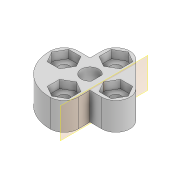
# Autodesk Inventor part: sonic hub 1_4 D 3mm
Saved by Autodesk Inventor 2020 (Build 240168000, 168)
## iProperties
Created: 2019-12-14
Part Number: sonic hub 1_4 D 3mm
Material: Generic
Document SubType Name: Modeling
Designer: ball
Density: 1 g/cm^3
Appearance: Default
Author: ball
Autodesk Inventor part; units mm, degrees
ref_plane "YZ Plane" through (0, 0, 0) normal (1, 0, 0) x (0, 1, 0)
ref_plane "XZ Plane" through (0, 0, 0) normal (0, 1, 0) x (-1, 0, 0)
ref_plane "XY Plane" through (0, 0, 0) normal (0, 0, 1) x (1, 0, 0)
sketch "Sketch1" plane through (0, 0, 0) normal (0, 1, 0) x (-1, 0, 0)
  circle A0 centre (9.779, 0) radius 1.9304
  line L0 (0, 9.779) -> (0, 0) construction
  line L1 (9.779, 0) -> (0, 0) construction
  arc A1 (-2.5908, -2.0472) -> (-2.5908, 2.0472) centre (0, 0) ccw
  line L2 (-2.5908, 2.0472) -> (-2.5908, -2.0472)
  circle A2 centre (0, 9.779) radius 1.9304
  circle A3 centre (-9.779, 0) radius 1.9304
  circle A4 centre (0, -9.779) radius 1.9304
  line L3 (4.7625, 7.21) -> (-2.8575, 7.21) construction
  line L4 (-2.8575, 7.21) -> (-2.8575, 3.81) construction
  line L5 (-2.8575, 3.81) -> (4.7625, 3.81) construction
  line L6 (4.7625, 3.81) -> (4.7625, 7.21) construction
  line L7 (4.7625, 8.2835) -> (7.5625, 8.2835) construction
  line L8 (7.5625, 8.2835) -> (7.5625, 2.3835) construction
  line L9 (7.5625, 2.3835) -> (4.7625, 2.3835) construction
  line L10 (4.7625, 2.3835) -> (4.7625, 8.2835) construction
  circle A5 centre (0, -9.779) radius 5.2959 construction
  circle A6 centre (0, 9.779) radius 5.2959 construction
  circle A7 centre (9.779, 0) radius 5.2959 construction
  circle A8 centre (-9.779, 0) radius 5.2959 construction
  line L11 (-5.2959, 9.779) -> (-5.2959, -11.9726) construction
  line L12 (-9.779, 5.2959) -> (-5.2959, 5.2959)
  line L13 (-13.5238, -3.7448) -> (-3.7448, -13.5238)
  line L14 (5.2959, -9.779) -> (5.2959, 9.779) construction
  line L15 (9.779, -5.2959) -> (5.2959, -5.2959)
  line L16 (5.2959, -9.779) -> (5.2959, -5.2959)
  arc A9 (-9.779, 5.2959) -> (-13.5238, -3.7448) centre (-9.779, 0) ccw
  arc A10 (-3.7448, -13.5238) -> (5.2959, -9.779) centre (0, -9.779) ccw
  line L17 (-5.2959, 9.779) -> (-5.2959, 5.2959)
  arc A11 (15.0749, 0) -> (0, 15.0749) centre (0, 0) ccw
  arc A12 (0, 15.0749) -> (-5.2959, 9.779) centre (0, 9.779) ccw
  arc A13 (9.779, -5.2959) -> (15.0749, 0) centre (9.779, 0) ccw
  dimension "d0" = 3.8608
  dimension "d2" = 0
  dimension "d3" = 9.779
  dimension "d12" = 6.604
  dimension "d13" = 2.5908
  dimension "d16" = 360
  dimension "d18" = 7.62
  dimension "d19" = 3.4
  dimension "d20" = 3.81
  dimension "d21" = 2.8
  dimension "d22" = 5.9
  dimension "d23" = 10.5918
  dimension "d24" = 10.5918
  dimension "d25" = 10.5918
  dimension "d26" = 10.5918
  constraints: 36 end point, 22 point on circle, 14 centre point, 10 coincident, 8 tangent, 4 parallel, 4 perpendicular, 3 point on line, 3 vertical, 2 collinear, 2 concentric, 2 horizontal, 9 other
  measures "d0" diameter of A0
  measures "d2" vertical distance of L0.end A0.centre
  measures "d3" distance of L0.end A0.centre
  measures "d12" diameter of A1
  measures "d13" distance from line of L2 L0.end
  measures "d18" distance of L5.end L4.end
  measures "d19" distance of L4.end L3.end
  measures "d20" distance from line of L0.end L5
  measures "d21" distance of L8.end L9.end
  measures "d22" distance of L7.end L8.end
  measures "d23" diameter of A5
  measures "d24" diameter of A6
  measures "d25" diameter of A7
  measures "d26" diameter of A8
extrude "Extrusion1" add sketch "Sketch1" along normal mid plane 10.4
sketch "Sketch2" plane through (0, 5.2, 0) normal (0, 1, 0) x (1, 0, 0)
  circle A0 centre (-9.779, 0) radius 1.9304 construction
  circle A1 centre (-9.779, 0) radius 4.6609 construction
  line L0 (-14.4399, 0) -> (-12.1095, 4.0365)
  line L1 (-12.1095, 4.0365) -> (-7.4486, 4.0365)
  line L2 (-7.4486, 4.0365) -> (-5.1181, 0)
  line L3 (-5.1181, 0) -> (-7.4485, -4.0365)
  line L4 (-7.4485, -4.0365) -> (-12.1094, -4.0365)
  line L5 (-12.1094, -4.0365) -> (-14.4399, 0)
  circle A2 centre (0, -9.779) radius 4.6609 construction
  line L6 (0, -14.4399) -> (-4.0365, -12.1095)
  line L7 (-4.0365, -12.1095) -> (-4.0365, -7.4486)
  line L8 (-4.0365, -7.4486) -> (0, -5.1181)
  line L9 (0, -5.1181) -> (4.0365, -7.4485)
  line L10 (4.0365, -7.4485) -> (4.0365, -12.1094)
  line L11 (4.0365, -12.1094) -> (0, -14.4399)
  circle A3 centre (9.779, 0) radius 4.6609 construction
  line L12 (14.4399, 0) -> (12.1095, -4.0365)
  line L13 (12.1095, -4.0365) -> (7.4486, -4.0365)
  line L14 (7.4486, -4.0365) -> (5.1181, 0)
  line L15 (5.1181, 0) -> (7.4485, 4.0365)
  line L16 (7.4485, 4.0365) -> (12.1094, 4.0365)
  line L17 (12.1094, 4.0365) -> (14.4399, 0)
  circle A4 centre (0, 9.779) radius 4.6609 construction
  line L18 (0, 14.4399) -> (4.0365, 12.1095)
  line L19 (4.0365, 12.1095) -> (4.0365, 7.4485)
  line L20 (4.0365, 7.4485) -> (0, 5.1181)
  line L21 (0, 5.1181) -> (-4.0365, 7.4485)
  line L22 (-4.0365, 7.4485) -> (-4.0365, 12.1094)
  line L23 (-4.0365, 12.1094) -> (0, 14.4399)
  point P0 (0, 0)
  dimension "d29" = 9.3218
  dimension "d32" = 360
  constraints: 48 end point, 8 coincident, 2 horizontal alignment, 2 vertical alignment, 86 other
extrude "Extrusion2" cut sketch "Sketch2" against normal blind 3.048
ref_plane "Work Plane1" through (5.2959, 0, 9.779) normal (1, 0, 0) x (0, 1, 0)
sketch "Sketch3" plane through (5.2959, 0, 9.779) normal (1, 0, 0) x (0, 1, 0)
  line L0 (2.152, -1.9304) -> (-5.2, -1.9304) construction
  line L1 (5.2, -6.477) -> (-5.2, -6.477) construction
  point P0 (0, -9.779)
  point P1 (0, -4.2037)
  dimension "d36" = 4.5466
  dimension "d37" = 2.2733
  measures "d36" distance between parallel lines of L1 L0
  measures "d37" distance from line of L0 point (0, -4.204)
hole "Hole1" [suppressed]
sketch "Sketch4" plane through (5.2959, 0, 9.779) normal (1, 0, 0) x (0, 1, 0)
  circle A0 centre (0, -4.2037) radius 1.7 projected
  circle A1 centre (0, -4.2037) radius 2.95
  point P0 (0, -9.779)
  dimension "d45" = 5.9
  constraints: 1 centre point, 1 coincident
  measures "d45" diameter of A1
extrude "Extrusion3" [suppressed]
sketch "Sketch5" plane through (0, -5.2, 0) normal (0, -1, 0) x (1, 0, 0)
  point P0 (0, 0)
equation "\"d23\" = d24"
equation "\"d25\" = d24"
equation "\"d26\" = d24"
equation "\"d37\" = 0.5 * d36"
body "Solid1"
